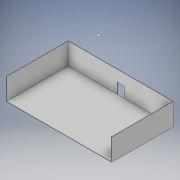
# Autodesk Inventor part: Top Office Layer
Saved by Autodesk Inventor 2017 (Build 210142000, 142)
## iProperties
Created: 2018-04-13
Part Number: Top Office Layer
Material: Generic
Document SubType Name: Modeling
Designer: landontracy
Density: 1 g/cm^3
Appearance: Default
Author: landontracy
Autodesk Inventor part; units mm, degrees
ref_plane "YZ Plane" through (0, 0, 0) normal (1, 0, 0) x (0, 1, 0)
ref_plane "XZ Plane" through (0, 0, 0) normal (0, 1, 0) x (-1, 0, 0)
ref_plane "XY Plane" through (0, 0, 0) normal (0, 0, 1) x (1, 0, 0)
sketch "Sketch1" plane through (0, 0, 0) normal (0, 0, 1) x (1, 0, 0)
  line L0 (73.602, -5752.0598) -> (12773.602, -5752.0598)
  line L1 (12773.602, -5752.0598) -> (12773.602, -12102.0598)
  line L2 (73.602, -12102.0598) -> (73.602, -5752.0598)
  line L3 (12773.602, -12102.0598) -> (8328.602, -12102.0598)
  line L4 (4518.602, -12102.0598) -> (73.602, -12102.0598)
  line L5 (5471.102, -8927.0598) -> (7607.6193, -8927.0598)
  line L6 (7607.6193, -8927.0598) -> (7607.6193, -12102.0598)
  line L7 (5471.102, -12102.0598) -> (5471.102, -8927.0598)
  line L8 (4518.602, -12102.0598) -> (5471.102, -12102.0598)
  line L9 (7607.6193, -12102.0598) -> (8328.602, -12102.0598)
  point P0 (0, 0)
  dimension "d0" = 12700
  dimension "d1" = 6350
  constraints: 20 end point, 4 parallel, 3 horizontal, 2 perpendicular, 1 collinear
  measures "d0" distance of L1.end L2.start
  measures "d1" distance of L0.end L1.end
sketch "Sketch2" plane through (0, 0, 0) normal (0, 0, 1) x (1, 0, 0)
  point P0 (0, 0)
extrude "Extrusion1" add sketch "Sketch1" along normal blind 127
sketch "Sketch3" plane through (0, 0, 127) normal (0, 0, 1) x (1, 0, 0)
  point P0 (0, 0)
sketch "Sketch4" plane through (0, 0, 127) normal (0, 0, 1) x (1, 0, 0)
  point P0 (0, 0)
sketch "Sketch5" plane through (73.602, -12102.0598, 0) normal (-1, 0, 0) x (0, 0, 1)
  line L0 (127, 3891.009) -> (127, 0) projected
  line L1 (0, 6350) -> (127, 6350)
  line L2 (127, 6350) -> (127, 0)
  line L3 (127, 0) -> (0, 0)
  line L4 (0, 0) -> (0, 6350)
  point P0 (0, 12102.0598)
  constraints: 8 end point, 2 parallel, 1 horizontal, 1 perpendicular
extrude "Extrusion2" add sketch "Sketch5" along normal blind 8890
sketch "Sketch6" plane through (12773.602, -12102.0598, 0) normal (1, 0, 0) x (0, 0, -1)
  line L0 (-127, 0) -> (-127, 6350) projected
  line L1 (0, 0) -> (-127, 0) projected
  line L2 (-127, 6350) -> (0, 6350)
  line L3 (0, 6350) -> (0, 0)
  line L4 (0, 0) -> (-127, 0)
  line L5 (-127, 0) -> (-127, 6350)
  point P0 (0, 12102.0598)
  constraints: 8 end point, 2 parallel, 1 horizontal, 1 perpendicular
extrude "Extrusion3" add sketch "Sketch6" along normal blind 8890
sketch "Sketch7" plane through (0, 0, 127) normal (0, 0, 1) x (1, 0, 0)
  line L0 (5471.102, -12102.0598) -> (-8816.398, -12102.0598) projected
  line L1 (21663.602, -5752.0598) -> (21663.602, -12102.0598) projected
  line L2 (-8816.398, -12102.0598) -> (21663.602, -12102.0598)
  line L3 (21663.602, -12102.0598) -> (21663.602, -11975.0598)
  line L4 (21663.602, -11975.0598) -> (-8816.398, -11975.0598)
  line L5 (-8816.398, -11975.0598) -> (-8816.398, -12102.0598)
  point P0 (0, 0)
  point P1 (4518.602, -12102.0598)
  dimension "d9" = 127
  constraints: 8 end point, 2 parallel, 1 horizontal, 1 perpendicular, 1 point on line
  measures "d9" distance of L3.end L2.end
extrude "Extrusion4" add sketch "Sketch7" along normal blind 17780
sketch "Sketch8" plane through (0, 0, 127) normal (0, 0, 1) x (1, 0, 0)
  line L0 (-8816.398, -5752.0598) -> (-8816.398, -12102.0598) projected
  line L1 (-8816.398, -11975.0598) -> (5471.102, -11975.0598) projected
  line L2 (-8816.398, -5752.0598) -> (-8689.398, -5752.0598)
  line L3 (-8689.398, -5752.0598) -> (-8689.398, -11975.0598)
  line L4 (-8689.398, -11975.0598) -> (-8816.398, -11975.0598)
  line L5 (-8816.398, -11975.0598) -> (-8816.398, -5752.0598)
  line L6 (4518.602, -8211.0508) -> (8328.602, -8211.0508) projected
  line L7 (6423.602, -8211.0508) -> (6423.602, -9947.683)
  line L8 (21663.602, -5752.0598) -> (21663.602, -12102.0598)
  line L9 (21663.602, -11975.0598) -> (8328.602, -11975.0598)
  line L10 (21663.602, -5752.0598) -> (21536.602, -5752.0598)
  line L11 (21536.602, -5752.0598) -> (21536.602, -11975.0598)
  point P0 (0, 0)
  point P1 (4518.602, -11975.0598)
  dimension "d12" = 127
  constraints: 18 end point, 6 symmetric about line, 2 parallel, 2 point on line, 1 horizontal, 1 midpoint, 1 perpendicular, 1 vertical
  measures "d12" distance of L3.end L4.end
extrude "Extrusion5" add sketch "Sketch8" along normal blind 17780 contours L2 L3 L1 L0
sketch "Sketch9" plane through (0, 0, 127) normal (0, 0, 1) x (1, 0, 0)
  line L0 (-8816.398, -5752.0598) -> (21663.602, -5752.0598) projected
  line L1 (21663.602, -5752.0598) -> (21536.602, -5752.0598)
  line L2 (21536.602, -5752.0598) -> (21536.602, -11979.2146)
  line L3 (21536.602, -11979.2146) -> (21663.602, -11979.2146)
  line L4 (21663.602, -11979.2146) -> (21663.602, -5752.0598)
  point P0 (0, 0)
  dimension "d15" = 127
  constraints: 8 end point, 2 parallel, 1 horizontal, 1 perpendicular
  measures "d15" distance of L3.end L2.end
extrude "Extrusion6" add sketch "Sketch9" along normal blind 17780
body "Solid1"
